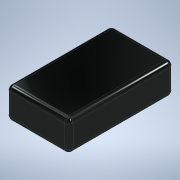
# Autodesk Inventor part: Driver
Saved by Autodesk Inventor 2021 (Build 250183000, 183)
## iProperties
Created: 2022-02-02
Part Number: Driver
Material: Generic
Document SubType Name: Modeling
Designer: deuts
Density: 1 g/cm^3
Appearance: Default
Author: deuts
Autodesk Inventor part; units mm, degrees
ref_plane "YZ Plane" through (0, 0, 0) normal (1, 0, 0) x (0, 1, 0)
ref_plane "XZ Plane" through (0, 0, 0) normal (0, 1, 0) x (-1, 0, 0)
ref_plane "XY Plane" through (0, 0, 0) normal (0, 0, 1) x (1, 0, 0)
sketch "Sketch1" plane through (0, 0, 0) normal (0, 1, 0) x (-1, 0, 0)
  line L0 (-28.5, 48) -> (28.5, 48)
  line L1 (28.5, 48) -> (28.5, -48)
  line L2 (28.5, -48) -> (-28.5, -48)
  line L3 (-28.5, -48) -> (-28.5, 48)
  line L4 (-28.5, 48) -> (28.5, -48) construction
  line L5 (28.5, 48) -> (-28.5, -48) construction
  point P0 (0, 0)
  dimension "d0" = 57
  dimension "d1" = 96
  constraints: 12 end point, 2 midpoint, 2 parallel, 1 horizontal, 1 perpendicular
  measures "d0" distance of L1.end L2.end
  measures "d1" distance of L0.end L1.end
extrude "Extrusion1" add sketch "Sketch1" along normal blind 28
fillet "Fillet1" radius 4 12 edges at (28.5, 14, 48) (28.5, 14, -48) (28.5, 28, 0) (28.5, 0, 0) (0, 28, -48) (-28.5, 28, 0) (0, 28, 48) (0, 0, 48) (-28.5, 0, 0) (-28.5, 14, 48) (-28.5, 14, -48) (0, 0, -48)
body "Solid1"
